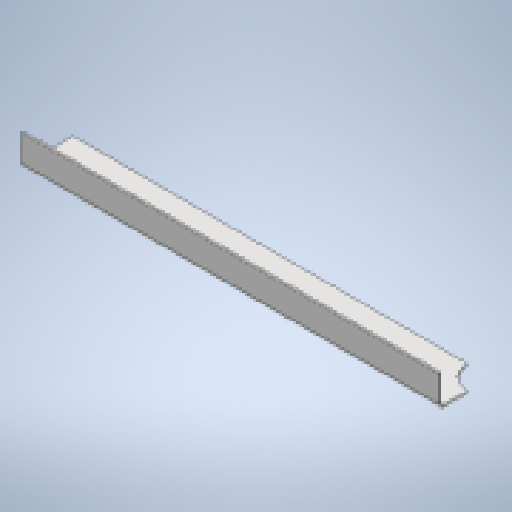
# Autodesk Inventor part: MSC 068 stringer lowerback
Saved by Autodesk Inventor 2025 (Build 290162010, 162A)
## iProperties
Created: 2024-04-28
Part Number: MSC 068 stringer lowerback
Material: Stainless Steel
Document SubType Name: Sheet Metal
Designer: admin
Stock Number: МОО 068 стрингер поясница
Density: 8 g/cm^3
Flat Pattern Width: 65 cm
Flat Pattern Length: 7.6202 cm
Flat Pattern Area: 495.313 cm^2
Sheet Metal Rule: AISI304 2mm Die16
Sheet Metal Width: 650,000 mm
Sheet Metal Length: 76,202 mm
Sheet Metal Area: 49531,294 mm^2
Appearance: Default
Author: admin
Autodesk Inventor part; units mm, degrees
ref_plane "YZ Plane" through (0, 0, 0) normal (1, 0, 0) x (0, 1, 0)
ref_plane "XZ Plane" through (0, 0, 0) normal (0, 1, 0) x (-1, 0, 0)
ref_plane "XY Plane" through (0, 0, 0) normal (0, 0, 1) x (1, 0, 0)
sketch "Sketch1" plane through (0, 0, 0) normal (0, 0, 1) x (1, 0, 0)
  line L0 (-650, 50) -> (0, 50)
  line L1 (0, 50) -> (0, 0)
  line L2 (0, 0) -> (-650, 0)
  line L3 (-650, 0) -> (-650, 50)
  point P0 (-325, 0)
  dimension "d1" = 50
  dimension "d45" = 650
  measures "d1" distance of L0.end L1.end
  measures "d45" distance of L1.end L2.end
extrude "Plate1" add sketch "Sketch1" along normal blind 2
sketch "Sketch2" plane through (0, 2, 0) normal (0, -1, 0) x (1, 0, 0)
  line L0 (-650, 0) -> (0, 0)
  line L1 (0, 0) -> (0, 30)
  line L2 (0, 30) -> (-650, 30)
  line L3 (-650, 30) -> (-650, 0)
  constraints: 6 end point, 1 horizontal, 1 perpendicular, 1 vertical
edge flange "Flange1" height 30 angle 90 thickness 2 bend radius 2.75 thickness toward (0, -1, 0) relief round relief width 2 relief depth 1 edges at (-325, 0, 2) wall of the first edge with corners at (-650, 2, 0) (0, 2, 0) (0, 2, 30) (-650, 2, 30)
bend "Bend1"
corner "Corner1"
sketch "Sketch6" plane through (0, 0, 0) normal (0, 0, -1) x (-1, 0, 0)
  line L0 (0, 50) -> (0, 4.75) projected
  circle A0 centre (0, 50) radius 22.5
  line L1 (0, 50) -> (650, 50) projected
  line L2 (-1, 67.6691) -> (-1, 30) projected
  line L3 (-499, 30) -> (-499, 67.6691) projected
  line L4 (-1, 30) -> (-499, 30) construction
  circle A1 centre (-250, 50) radius 22.5
  point P0 (0, 0)
  point P1 (22.5, 50)
  point P2 (0, 27.5)
  point P3 (-250, 30)
  dimension "d24" = 45
  constraints: 2 centre point, 2 end point, 1 equal radius, 1 midpoint, 1 perpendicular, 1 vertical alignment, 2 other
  measures "d24" diameter of A0
extrude "Extrusion2" cut sketch "Sketch6" along normal mid plane 30 contours L1 A0 L0 picked at (14.812, 48.3311)
sketch "Sketch7" plane through (0, 0, 2) normal (0, 0, 1) x (1, 0, 0)
  line L0 (-650, 4.75) -> (-650, 50) projected
  line L1 (-650, 4.75) -> (0, 4.75) projected
  line L2 (0, 27.5) -> (0, 4.75) projected
  arc A0 (-22.5, 50) -> (0, 27.5) centre (0, 50) ccw projected
  line L3 (-650, 50) -> (-22.5, 50) projected
  line L4 (-101, 23.375) -> (-99, 23.375)
  line L5 (-99, 23.375) -> (-99, 31.375)
  line L6 (-99, 31.375) -> (-101, 31.375)
  line L7 (-101, 31.375) -> (-101, 23.375)
  line L8 (-650, 4.75) -> (0, 4.75) projected
  line L9 (-100, 4.75) -> (-100, 50) construction
  line L10 (-113, 23.375) -> (-111, 23.375)
  line L11 (-111, 23.375) -> (-111, 31.375)
  line L12 (-111, 31.375) -> (-113, 31.375)
  line L13 (-113, 31.375) -> (-113, 23.375)
  point P0 (0, 0)
  point P1 (-100, 23.375)
  point P2 (-101, 27.375)
  point P3 (-100, 27.375)
  point P4 (-111, 27.375)
  dimension "d30" = 2
  dimension "d31" = 8
  dimension "d32" = 100
  dimension "d33" = 2
  dimension "d34" = 8
  dimension "d35" = 10
  constraints: 18 end point, 4 midpoint, 4 parallel, 3 perpendicular, 2 horizontal, 2 horizontal alignment, 2 point on line, 1 vertical alignment
  measures "d30" distance of L6.end L5.end
  measures "d31" distance of L5.end L4.end
  measures "d32" distance from line of L2 L9.end
  measures "d33" distance of L12.end L11.end
  measures "d34" distance of L11.end L10.end
  measures "d35" distance of L4.start L10.end
extrude "Extrusion3" [suppressed]
mirror "Mirror2" [suppressed]
sketch "Sketch9" plane through (0, 0, 2) normal (0, 0, 1) x (1, 0, 0)
  line L0 (494, 45) -> (494, 33) construction
  line L1 (494, 33) -> (294, 33) construction
  line L2 (294, 33) -> (294, 45) construction
  line L3 (294, 45) -> (494, 45) construction
  line L4 (499, 30) -> (499, 67.6691) projected
  line L5 (-650, 50) -> (0, 50) projected
  point P0 (0, 0)
  point P1 (1, 67.6691)
  point P2 (0, 50)
  dimension "d40" = 200
  dimension "d41" = 12
  dimension "d42" = 5
  dimension "d43" = 5
  constraints: 3 other
  measures "d40" distance of L0.end L1.end
  measures "d41" distance of L1.end L2.end
  measures "d42" distance between parallel lines of L4 L0
feature "Mark2" [suppressed]
equation "\"d43\" = d42"
equation "\"d2\" = Thickness"
equation "\"d3\" = BendReliefWidth"
equation "\"d4\" = BendReliefDepth"
equation "\"d5\" = MinimumRemnant"
equation "\"d6\" = TransitionRadius"
equation "\"d9\" = BendRadius"
equation "\"d10\" = CornerReliefSize"
equation "\"d11\" = GapSize"
equation "\"d12\" = JacobiRadiusSize"
equation "\"BendReliefWidth\" = Thickness"
equation "\"BendReliefDepth\" = 0.5 * Thickness"
equation "\"CornerReliefSize\" = 4 * Thickness"
equation "\"MinimumRemnant\" = 2 * Thickness"
equation "\"TransitionRadius\" = BendRadius"
equation "\"JacobiRadiusSize\" = BendRadius"
equation "\"GapSize\" = Thickness"
equation "\"qqqqqq\" = 67.35706"
equation "\"Thickness\" = 2"
equation "\"BendRadius\" = 2.75"
body "Solid1"
